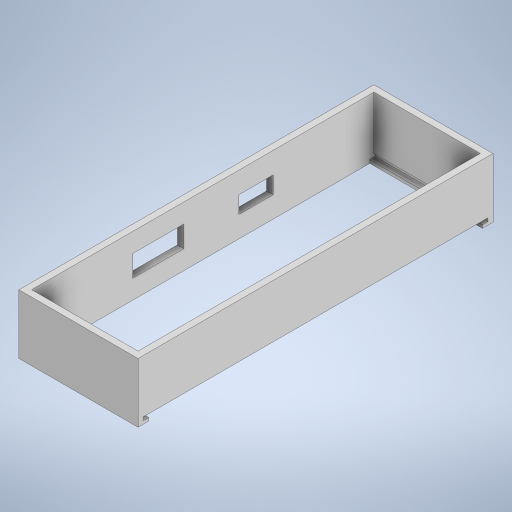
# Autodesk Inventor part: Part1
Saved by Autodesk Inventor 2024 (Build 280153000, 153)
## iProperties
Created: 2025-02-26
Part Number: Part1
Material: Generic
Document SubType Name: Modeling
Designer: vandevelde.wout
Density: 1 g/cm^3
Appearance: Default
Author: vandevelde.wout
Autodesk Inventor part; units mm, degrees
ref_plane "YZ Plane" through (0, 0, 0) normal (1, 0, 0) x (0, 1, 0)
ref_plane "XZ Plane" through (0, 0, 0) normal (0, 1, 0) x (-1, 0, 0)
ref_plane "XY Plane" through (0, 0, 0) normal (0, 0, 1) x (1, 0, 0)
sketch "Sketch1" plane through (0, 0, 0) normal (0, 1, 0) x (-1, 0, 0)
  line L0 (0, 0) -> (50, 0)
  line L1 (50, 0) -> (50, -161)
  line L2 (50, -161) -> (0, -161)
  line L3 (0, -161) -> (0, 0)
  line L4 (0, 0) -> (-3, 0)
  line L5 (-3, 0) -> (-3, 3)
  line L6 (-3, 3) -> (53, 3)
  line L7 (53, 3) -> (53, -164)
  line L8 (53, -164) -> (-3, -164)
  line L9 (-3, -164) -> (-3, 0)
  dimension "d0" = 50
  dimension "d1" = 161
  dimension "d2" = 3
  dimension "d3" = 3
  dimension "d4" = 56
  dimension "d5" = 167
  dimension "d6" = 56
  constraints: 20 end point, 5 perpendicular, 2 parallel, 1 collinear, 1 horizontal, 1 point on line
  measures "d0" distance of L1.end L2.end
  measures "d1" distance of L0.end L1.end
  measures "d2" distance of L0.start L4.end
  measures "d3" distance of L4.end L5.end
  measures "d4" distance of L5.end L6.end
  measures "d5" distance of L6.end L7.end
  measures "d6" distance of L7.end L8.end
extrude "Extrusion1" add sketch "Sketch1" along normal blind 25
sketch "Sketch2" plane through (3, 0, 3) normal (1, 0, 0) x (0, 0, -1)
  line L0 (0, 0) -> (0, 25) projected
  line L1 (0, 0) -> (0, -3)
  line L2 (0, -3) -> (5, -3)
  line L3 (5, -3) -> (5, -1.5)
  line L4 (5, -1.5) -> (2.5, -1.5)
  line L5 (2.5, -1.5) -> (2.5, 0)
  line L6 (0, 0) -> (167, 0) projected
  line L7 (167, 0) -> (167, -3)
  line L8 (167, -3) -> (162, -3)
  line L9 (162, -3) -> (162, -1.5)
  line L10 (162, -1.5) -> (164.5, -1.5)
  line L11 (164.5, -1.5) -> (164.5, 0)
  point P0 (3, 0)
  dimension "d9" = 3
  dimension "d10" = 5
  dimension "d11" = 1.5
  dimension "d12" = 2.5
  dimension "d13" = 3
  dimension "d14" = 5
  dimension "d15" = 1.5
  dimension "d16" = 2.5
  constraints: 20 end point, 7 perpendicular, 2 vertical, 1 horizontal
  measures "d9" distance of L0.start L1.end
  measures "d10" distance of L1.end L2.end
  measures "d11" distance of L2.end L3.end
  measures "d12" distance of L3.end L4.end
  measures "d13" distance of L6.end L7.end
  measures "d14" distance of L7.end L8.end
  measures "d15" distance of L8.end L9.end
  measures "d16" distance of L9.end L10.end
extrude "Extrusion2" add sketch "Sketch2" against normal blind 56
sketch "Sketch3" plane through (3, 25, -164) normal (0, 0, -1) x (-1, 0, 0)
  line L0 (0, -28) -> (56, -28) projected
  line L1 (56, -28) -> (56, -25)
  line L2 (56, -28) -> (56, 0) projected
  line L3 (56, -25) -> (53, -25)
  line L4 (53, -25) -> (53, -28)
  line L5 (53, -28) -> (56, -28)
  point P0 (3, -25)
  dimension "d19" = 3
  dimension "d20" = 3
  constraints: 8 end point, 3 perpendicular, 1 point on line
  measures "d19" distance of L0.end L1.end
  measures "d20" distance of L1.end L3.end
extrude "Extrusion3" add sketch "Sketch3" against normal blind 167
sketch "Sketch4" plane through (3, 25, -164) normal (0, 0, -1) x (-1, 0, 0)
  point P0 (3, -25)
sketch "Sketch6" plane through (-53, 25, -164) normal (-1, 0, 0) x (0, 0, 1)
  line L0 (92.5, -9) -> (116.5, -9)
  line L1 (116.5, -9) -> (116.5, -19)
  line L2 (116.5, -19) -> (92.5, -19)
  line L3 (92.5, -19) -> (92.5, -9)
  line L4 (167, -28) -> (167, 0) projected
  line L5 (0, -28) -> (0, 0) projected
  line L6 (0, 0) -> (167, 0) projected
  line L7 (0, -28) -> (167, -28) projected
  point P0 (164, -25)
  point P1 (167, -14)
  dimension "d29" = 74.5
  dimension "d30" = 116.5
  dimension "d31" = 10
  dimension "d32" = 9
  dimension "d33" = 9
  constraints: 8 end point, 2 parallel, 1 horizontal, 1 midpoint, 1 perpendicular
  measures "d29" distance from line of point (167, -14) L3
  measures "d30" distance between parallel lines of L5 L1
  measures "d31" distance between parallel lines of L2 L0
  measures "d32" distance between parallel lines of L6 L0
  measures "d33" distance between parallel lines of L7 L2
extrude "Extrusion5" cut sketch "Sketch6" against normal blind 10 contours L0 L1 L2 L3
sketch "Sketch7" plane through (-53, 25, -164) normal (-1, 0, 0) x (0, 0, 1)
  line L0 (167, -28) -> (167, 0) projected
  line L1 (116.5, -9) -> (116.5, -19) projected
  line L2 (50.5, -10) -> (66.5, -10)
  line L3 (66.5, -10) -> (66.5, -18)
  line L4 (66.5, -18) -> (50.5, -18)
  line L5 (50.5, -18) -> (50.5, -10)
  line L6 (50.5, -10) -> (66.5, -18) construction
  line L7 (66.5, -10) -> (50.5, -18) construction
  line L8 (0, -28) -> (0, 0) projected
  line L9 (0, 0) -> (167, 0) projected
  point P0 (164, -25)
  point P1 (58.5, -14)
  dimension "d36" = 50.5
  dimension "d37" = 16
  dimension "d38" = 8
  dimension "d39" = 50.5
  dimension "d40" = 10
  constraints: 12 end point, 2 midpoint, 2 parallel, 1 horizontal, 1 perpendicular
  measures "d36" distance between parallel lines of L0 L1
  measures "d37" distance of L3.end L4.end
  measures "d38" distance of L2.end L3.end
  measures "d39" distance between parallel lines of L8 L5
  measures "d40" distance between parallel lines of L9 L2
extrude "Extrusion6" cut sketch "Sketch7" against normal blind 10
body "Solid1"
